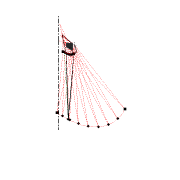
# Autodesk Inventor part: COXA_YAW_SERVO_BASE
Saved by Autodesk Inventor 2019.4 (Build 234330000, 330)
## iProperties
Created: 2019-10-21
Part Number: COXA_YAW_SERVO_BASE
Material: 一般
Document SubType Name: Modeling
Designer: y6tada
Density: 1 g/cm^3
Appearance: Black 80
Author: y6tada
Autodesk Inventor part; units mm, degrees
ref_plane "YZ Plane" through (0, 0, 0) normal (1, 0, 0) x (0, 1, 0)
ref_plane "XZ Plane" through (0, 0, 0) normal (0, 1, 0) x (-1, 0, 0)
ref_plane "XY Plane" through (0, 0, 0) normal (0, 0, 1) x (1, 0, 0)
sketch "スケッチ1" plane through (0, 0, 0) normal (0, 0, 1) x (1, 0, 0)
  line L0 (55.9065, 0) -> (6, 70) construction
  line L1 (55.9065, 0) -> (71, -21.1704)
  line L2 (71, -21.1704) -> (35, -35.0321)
  line L3 (0, 0) -> (0, 100.9173)
  line L4 (0, 0) -> (55.9065, 0) construction
  arc A0 (21.0922, 34.0034) -> (18.6986, 23.8341) centre (62.4221, 18.9089) ccw construction
  arc A1 (13.5777, 36.7479) -> (10.7489, 24.7295) centre (62.4221, 18.9089) ccw construction
  arc A2 (10.7489, 24.7295) -> (18.6986, 23.8341) centre (14.7237, 24.2818) ccw construction
  line L5 (14.7237, 24.2818) -> (62.4221, 18.9089) construction
  line L6 (62.4221, 18.9089) -> (16.3697, 32.4431)
  arc A3 (16.3697, 32.4431) -> (14.7237, 24.2818) centre (62.4221, 18.9089) ccw construction
  line L7 (14.7237, 24.2818) -> (69.8724, -18.83) construction
  line L8 (69.8724, -18.83) -> (72.9641, 19.6224) construction
  line L9 (16.3697, 32.4431) -> (35, -35.0321)
  line L10 (16.3697, 32.4431) -> (6, 70) construction
  line L11 (16.3697, 32.4431) -> (55.9065, 0) construction
  arc A4 (58.1726, -25.9011) -> (72.9641, 19.6224) centre (55.9065, 0) ccw
  line L12 (35, -35.0321) -> (71, -35.0321) construction
  line L13 (71, -35.0321) -> (71, -21.1704) construction
  line L14 (28.1647, -35.0321) -> (45, -295.0321) construction
  line L15 (55.9065, 0) -> (54.4287, -2.6107)
  line L16 (55.9065, 0) -> (53.3085, -1.5) construction
  arc A5 (53.3085, -1.5) -> (58.7903, -0.8269) centre (55.9065, 0) ccw construction
  line L17 (55.9065, 0) -> (53.851, -2.1851) construction
  line L18 (55.9065, 0) -> (54.5679, -2.6848) construction
  line L19 (55.9065, 0) -> (55.3985, -2.9567) construction
  line L20 (55.9065, 0) -> (56.2721, -2.9776) construction
  line L21 (55.9065, 0) -> (57.1148, -2.7459) construction
  line L22 (55.9065, 0) -> (57.8549, -2.2812) construction
  line L23 (55.9065, 0) -> (58.4296, -1.6229) construction
  line L24 (55.9065, 0) -> (58.7903, -0.8269) construction
  line L25 (62.4221, 18.9089) -> (54.4287, -2.6107)
  line L26 (53.3085, -1.5) -> (62.4221, 18.9089) construction
  line L27 (62.4221, 18.9089) -> (58.7903, -0.8269) construction
  line L28 (56.6038, -7.9696) -> (58.1726, -25.9011) construction
  line L29 (58.871, -7.4305) -> (65.541, -24.149) construction
  line L30 (60.8866, -6.2609) -> (72.0919, -20.3478) construction
  line L31 (62.4797, -4.56) -> (77.2694, -14.8199) construction
  line L32 (63.515, -2.4721) -> (80.634, -8.0344) construction
  line L33 (63.9046, -0.1745) -> (81.9003, -0.5672) construction
  line L34 (63.6156, 2.1379) -> (80.9609, 6.9482) construction
  line L35 (62.6724, 4.2689) -> (77.8955, 13.874) construction
  line L36 (61.155, 6.0377) -> (72.9641, 19.6224) construction
  arc A6 (56.6038, -7.9696) -> (61.155, 6.0377) centre (55.9065, 0) ccw construction
  line L37 (17.335, 35.3757) -> (62.4221, 18.9089) construction
  arc A7 (17.335, 35.3757) -> (16.3697, 32.4431) centre (62.4221, 18.9089) ccw construction
  arc A8 (21.0922, 34.0034) -> (13.5777, 36.7479) centre (17.335, 35.3757) ccw construction
  line L38 (53.851, -2.1851) -> (62.4221, 18.9089) construction
  line L39 (62.4221, 18.9089) -> (16.8008, 33.832) construction
  line L40 (16.2787, 32.1295) -> (62.4221, 18.9089) construction
  line L41 (54.5679, -2.6848) -> (62.4221, 18.9089) construction
  line L42 (17.335, 35.3757) -> (20.5779, -34.5492) construction
  line L43 (20.5779, -34.5492) -> (58.1726, -25.9011) construction
  line L44 (16.8008, 33.832) -> (28.5726, -35.1711) construction
  line L45 (28.5726, -35.1711) -> (65.541, -24.149) construction
  line L46 (35, -35.0321) -> (45, -295.0321)
  line L47 (71, -21.1704) -> (45, -295.0321)
  line L48 (28.5726, -35.1711) -> (18.3365, -295.1619) construction
  line L49 (18.3365, -295.1619) -> (65.541, -24.149) construction
  line L50 (58.1726, -25.9011) -> (-6.1756, -293.3623) construction
  line L51 (-6.1756, -293.3623) -> (20.5779, -34.5492) construction
  line L52 (62.4221, 18.9089) -> (15.8092, 30.365) construction
  line L53 (62.4221, 18.9089) -> (15.4185, 28.6386) construction
  line L54 (62.4221, 18.9089) -> (15.1184, 27.055) construction
  line L55 (62.4221, 18.9089) -> (14.9084, 25.7246) construction
  line L56 (62.4221, 18.9089) -> (14.7803, 24.7619) construction
  line L57 (62.4221, 18.9089) -> (55.3985, -2.9567) construction
  line L58 (62.4221, 18.9089) -> (56.2721, -2.9776) construction
  line L59 (62.4221, 18.9089) -> (57.1148, -2.7459) construction
  line L60 (62.4221, 18.9089) -> (57.8549, -2.2812) construction
  line L61 (62.4221, 18.9089) -> (58.4296, -1.6229) construction
  line L62 (16.2787, 32.1295) -> (36.3751, -34.9237) construction
  line L63 (36.3751, -34.9237) -> (72.0919, -20.3478) construction
  line L64 (77.2694, -14.8199) -> (43.7056, -33.8362) construction
  line L65 (43.7056, -33.8362) -> (15.8092, 30.365) construction
  line L66 (15.4185, 28.6386) -> (50.4001, -31.9939) construction
  line L67 (50.4001, -31.9939) -> (80.634, -8.0344) construction
  line L68 (81.9003, -0.5672) -> (56.3772, -29.4932) construction
  line L69 (56.3772, -29.4932) -> (15.1184, 27.055) construction
  line L70 (14.9084, 25.7246) -> (61.6068, -26.4219) construction
  line L71 (61.6068, -26.4219) -> (80.9609, 6.9482) construction
  line L72 (77.8955, 13.874) -> (66.0919, -22.8523) construction
  line L73 (66.0919, -22.8523) -> (14.7803, 24.7619) construction
  line L74 (36.3751, -34.9237) -> (51.5513, -294.673) construction
  line L75 (72.9641, 19.6224) -> (308.5689, -122.3867) construction
  line L76 (308.5689, -122.3867) -> (69.8724, -18.83) construction
  line L77 (77.8955, 13.874) -> (274.7797, -178.2531) construction
  line L78 (274.7797, -178.2531) -> (66.0919, -22.8523) construction
  line L79 (61.6068, -26.4219) -> (232.4131, -222.7003) construction
  line L80 (232.4131, -222.7003) -> (80.9609, 6.9482) construction
  line L81 (81.9003, -0.5672) -> (185.3696, -255.46) construction
  line L82 (185.3696, -255.46) -> (56.3772, -29.4932) construction
  line L83 (50.4001, -31.9939) -> (137.422, -277.2023) construction
  line L84 (137.422, -277.2023) -> (80.634, -8.0344) construction
  line L85 (77.2694, -14.8199) -> (91.9175, -289.5228) construction
  line L86 (91.9175, -289.5228) -> (43.7056, -33.8362) construction
  line L87 (51.5513, -294.673) -> (72.0919, -20.3478) construction
  spline S0 degree 4 poles (-6.1756, -293.3623) (-10.5261, -296.2302) (59.5186, -294.0012) (28.5779, -297.1396) (108.8399, -288.6214) (137.581, -277.3672) (213.1132, -246.8036) (256.019, -203.8802) (293.9724, -158.7918) (308.5689, -122.3867) knots 0 0 0 0 0 0.206557 0.299066 0.400803 0.524642 0.654907 1 1 1 1 1 construction
  spline S1 degree 4 poles (20.5779, -34.5492) (25.4604, -35.1887) (32.3283, -35.5074) (40.838, -34.7864) (50.2408, -32.2372) (58.3828, -28.8709) (64.0234, -25.0643) (67.6552, -21.558) (69.8724, -18.83) knots 0 0 0 0 0 0.335047 0.464017 0.588993 0.710013 1 1 1 1 1
  circle A9 centre (62.4221, 18.9089) radius 4 construction
  line L88 (0, 0) -> (0, -360.2407)
  point P0 (55.9065, 0)
  point P1 (55.9065, 0)
  point P2 (55.9065, 0)
  point P3 (55.9065, 0)
  point P4 (55.9065, 0)
  point P5 (55.9065, 0)
  point P6 (55.9065, 0)
  point P7 (55.9065, 0)
  dimension "d5" = 70
  dimension "d66" = 26
  dimension "d67" = 36
  dimension "d74" = 65
  dimension "d76" = 3
  dimension "d80" = 134
  dimension "d82" = 20
  dimension "d85" = 134
  dimension "d87" = 65
  dimension "d88" = 70
  dimension "d89" = 86
  dimension "d90" = 86
  dimension "d91" = 86
  dimension "d92" = 4
  dimension "d93" = 86
  dimension "d94" = 86
  dimension "d95" = 95
  dimension "d96" = 86
  dimension "d97" = 86
  dimension "d98" = 86
  dimension "d99" = 86
  dimension "d100" = 86
  dimension "d101" = 8
  dimension "d102" = 6
  dimension "d104" = 72.448
  dimension "d105" = 8
  dimension "d106" = 84.427
  dimension "d111" = 13.8617
  dimension "d113" = 70
  dimension "d114" = 48
  dimension "d116" = 90
  dimension "d117" = 260
  constraints: 178 end point, 36 equal length, 28 point on circle, 17 coincident, 14 point on line, 10 centre point, 4 tangent, 2 horizontal, 2 vertical, 1 collinear, 1 concentric, 1 perpendicular, 76 other
  measures "d5" distance from line of L4 L0.end
  measures "d66" radius of A4
  measures "d67" distance of L2.end L12.end
  measures "d74" angle of L15 L1
  measures "d76" radius of A5
  measures "d82" distance of L0.start L5.end
  measures "d87" angle of L16 L28
  measures "d88" distance of L6.end L2.end
  measures "d89" angle of L25 L6
  measures "d90" angle of L26 L37
  measures "d91" angle of L27 L5
  measures "d92" radius of A8
  measures "d93" angle of L38 L39
  measures "d94" angle of L40 L41
  measures "d95" angle of L28 L4
  measures "d96" angle of L57 L52
  measures "d97" angle of L58 L53
  measures "d98" angle of L59 L54
  measures "d99" angle of L55 L60
  measures "d100" angle of L61 L56
  measures "d101" radius of A6
  measures "d102" distance from line of L0.end L3
  measures "d104" angle of L76 L51
  measures "d105" diameter of A9
  measures "d106" angle of L27 L24
  measures "d111" distance of L12.end L1.end
  measures "d113" diameter of L2.end L88
  measures "d114" distance of L5.end L6.end
  measures "d116" diameter of L14.end L88
  measures "d117" distance from line of L14.end L12
sketch "スケッチ2" plane through (0, 0, 0) normal (0, 0, 1) x (1, 0, 0)
  arc A0 (65.8862, 20.9089) -> (59.3619, 21.4848) centre (62.4221, 18.9089) ccw
  line L0 (40, 8) -> (64, 8) construction
  line L1 (64, 8) -> (64, -4) construction
  line L2 (64, -4) -> (40, -4) construction
  line L3 (40, -4) -> (40, 8) construction
  line L4 (36, 10.1673) -> (36, -48.9437) construction
  line L5 (67, 18.1759) -> (67, -4)
  line L6 (64, -7) -> (40, -7)
  line L7 (37, -4) -> (37, 8)
  arc A1 (37, -4) -> (40, -7) centre (40, -4) ccw
  arc A2 (39.6737, 10.9822) -> (37, 8) centre (40, 8) ccw
  arc A3 (64, -7) -> (67, -4) centre (64, -4) ccw
  line L8 (0, 0) -> (0, -59.5537) construction
  line L9 (10.6628, 2) -> (66.9205, 2) construction
  line L10 (66.5981, 19.6759) -> (65.8862, 20.9089)
  arc A4 (39.6737, 10.9822) -> (59.3619, 21.4848) centre (36.4106, 40.8042) ccw
  arc A5 (67, 18.1759) -> (66.5981, 19.6759) centre (64, 18.1759) ccw
  point P0 (67, 18.9798)
  dimension "d16" = 24
  dimension "d17" = 4
  dimension "d18" = 12
  dimension "d19" = 3
  dimension "d20" = 72
  dimension "d23" = 4
  dimension "d107" = 30
  dimension "d108" = 3
  dimension "d109" = 30
  dimension "d118" = 2
  constraints: 22 end point, 12 point on circle, 10 tangent, 6 centre point, 3 coincident, 3 horizontal, 3 parallel, 3 vertical, 2 equal radius, 2 point on line, 1 perpendicular, 1 other
  measures "d16" distance of L1.end L2.end
  measures "d17" distance between parallel lines of L3 L4
  measures "d18" distance of L2.end L0.start
  measures "d19" radius of A1
  measures "d20" diameter of L4 L8
  measures "d23" radius of A0
  measures "d107" radius of A4
  measures "d108" radius of A5
  measures "d109" angle of L5 L10
  measures "d118" distance from line of L9 L8.start
extrude "押し出し1" add sketch "スケッチ2" along normal blind 2
hole "穴1" at (62.4221, 18.9089, 0) direction (0, 0, 1) diameter 3 end through all
hole "穴2" at (64, 8, 0) at (40, 8, 0) at (40, -4, 0) at (64, -4, 0) direction (0, 0, 1) diameter 2.5 end through all
equation "\"input_link_length\" = 26"
equation "\"input_link_formed_angle\" = 65deg"
equation "\"support_formed_angle\" = 86deg"
equation "\"input_slider_radius\" = 3"
equation "\"driver_rotation_range\" = 134deg"
equation "\"virtual_mass_point_x\" = 6"
equation "\"driver_min_angle\" = 95deg"
equation "\"coupler_x\" = 36"
equation "\"support_link_length\" = 48"
